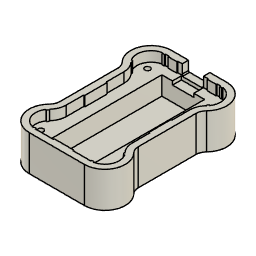
tiny-scarab-v0.2-enclosure (Autodesk Fusion 360 design; units mm, degrees)
Autodesk Fusion 360 part; units mm, degrees
sketch "board_cutout_1mm_offset" plane through (0, 0, 0) normal (0, 0, 1) x (1, 0, 0)
  line L0 (79.75, -21.495) -> (110.75, -21.495) construction
  arc A0 (79.75, -21.495) -> (74.3929, -34.2439) centre (79.75, -28.995) ccw construction
  arc A1 (77.25, -41.2424) -> (74.3929, -34.2439) centre (67.25, -41.2424) ccw construction
  line L1 (77.25, -41.2424) -> (77.25, -73.7476) construction
  arc A2 (74.3929, -80.7461) -> (77.25, -73.7476) centre (67.25, -73.7476) ccw construction
  arc A3 (74.3929, -80.7461) -> (79.75, -93.495) centre (79.75, -85.995) ccw construction
  line L2 (79.75, -93.495) -> (110.75, -93.495) construction
  arc A4 (110.75, -93.495) -> (116.1071, -80.7461) centre (110.75, -85.995) ccw construction
  arc A5 (113.25, -73.7476) -> (116.1071, -80.7461) centre (123.25, -73.7476) ccw construction
  line L3 (113.25, -41.2424) -> (113.25, -73.7476) construction
  arc A6 (116.1071, -34.2439) -> (113.25, -41.2424) centre (123.25, -41.2424) ccw construction
  arc A7 (116.1071, -34.2439) -> (110.75, -21.495) centre (110.75, -28.995) ccw construction
  arc A8 (76.75, -41.2424) -> (74.0357, -34.5938) centre (67.25, -41.2424) ccw
  arc A9 (78.3608, -21.1165) -> (73.1503, -33.5165) centre (79.75, -28.995) ccw
  arc A10 (117.3497, -33.5165) -> (112.1392, -21.1165) centre (110.75, -28.995) ccw
  arc A11 (116.4643, -34.5938) -> (113.75, -41.2424) centre (123.25, -41.2424) ccw
  arc A12 (113.75, -73.7476) -> (116.4643, -80.3962) centre (123.25, -73.7476) ccw
  arc A13 (112.1392, -93.8735) -> (117.3497, -81.4735) centre (110.75, -85.995) ccw
  arc A14 (73.1503, -81.4735) -> (78.3608, -93.8735) centre (79.75, -85.995) ccw
  arc A15 (74.0357, -80.3962) -> (76.75, -73.7476) centre (67.25, -73.7476) ccw
  line L4 (81.75, -20.995) -> (81.75, -21.495)
  line L5 (108.75, -21.495) -> (108.75, -20.995)
  line L6 (79.75, -20.995) -> (81.75, -20.995)
  line L7 (108.75, -20.995) -> (110.75, -20.995)
  line L8 (89.75, -93.995) -> (89.75, -93.495)
  line L9 (89.75, -93.495) -> (100.75, -93.495)
  line L10 (100.75, -93.495) -> (100.75, -93.995)
  line L11 (79.75, -93.995) -> (89.75, -93.995)
  line L12 (100.75, -93.995) -> (110.75, -93.995)
  line L13 (76.75, -51.2424) -> (77.25, -51.2424)
  line L14 (77.25, -51.2424) -> (77.25, -63.7476)
  line L15 (77.25, -63.7476) -> (76.75, -63.7476)
  line L16 (76.75, -41.2424) -> (76.75, -51.2424)
  line L17 (76.75, -63.7476) -> (76.75, -73.7476)
  line L18 (113.75, -51.2424) -> (113.25, -51.2424)
  line L19 (113.25, -51.2424) -> (113.25, -63.7476)
  line L20 (113.25, -63.7476) -> (113.75, -63.7476)
  line L21 (113.75, -41.2424) -> (113.75, -51.2424)
  line L22 (113.75, -63.7476) -> (113.75, -73.7476)
  line L23 (86.75, -21.495) -> (86.75, -20.995)
  line L24 (86.75, -20.995) -> (103.75, -20.995)
  line L25 (103.75, -20.995) -> (103.75, -21.495)
  line L26 (81.75, -21.495) -> (86.75, -21.495)
  line L27 (103.75, -21.495) -> (108.75, -21.495)
  arc A16 (116.1071, -34.2439) -> (116.9372, -33.2339) centre (110.75, -28.995) ccw
  line L28 (110.75, -28.995) -> (116.1071, -34.2439) construction
  line L29 (110.75, -28.995) -> (116.9372, -33.2339) construction
  line L30 (79.75, -28.995) -> (74.3929, -34.2439) construction
  arc A17 (73.5628, -33.2339) -> (74.3929, -34.2439) centre (79.75, -28.995) ccw
  line L31 (73.5628, -33.2339) -> (79.75, -28.995) construction
  line L32 (79.75, -85.995) -> (74.3929, -80.7461) construction
  arc A18 (74.3929, -80.7461) -> (73.5628, -81.7561) centre (79.75, -85.995) ccw
  line L33 (73.5628, -81.7561) -> (79.75, -85.995) construction
  line L34 (110.75, -85.995) -> (116.1071, -80.7461) construction
  arc A19 (116.9372, -81.7561) -> (116.1071, -80.7461) centre (110.75, -85.995) ccw
  line L35 (110.75, -85.995) -> (116.9372, -81.7561) construction
  line L36 (110.75, -85.995) -> (110.75, -93.495) construction
  arc A20 (110.75, -93.495) -> (112.0524, -93.3811) centre (110.75, -85.995) ccw
  line L37 (110.75, -85.995) -> (112.0524, -93.3811) construction
  line L38 (79.75, -85.995) -> (79.75, -93.495) construction
  arc A21 (78.4476, -93.3811) -> (79.75, -93.495) centre (79.75, -85.995) ccw
  line L39 (78.4476, -93.3811) -> (79.75, -85.995) construction
  line L40 (79.75, -28.995) -> (79.75, -21.495) construction
  arc A22 (79.75, -21.495) -> (78.4476, -21.6089) centre (79.75, -28.995) ccw
  line L41 (79.75, -28.995) -> (78.4476, -21.6089) construction
  line L42 (110.75, -28.995) -> (110.75, -21.495) construction
  arc A23 (112.0524, -21.6089) -> (110.75, -21.495) centre (110.75, -28.995) ccw
  line L43 (112.0524, -21.6089) -> (110.75, -28.995) construction
  line L44 (116.1071, -34.2439) -> (116.4643, -34.5938)
  line L45 (116.9372, -33.2339) -> (117.3497, -33.5165)
  line L46 (110.75, -21.495) -> (110.75, -20.995)
  line L47 (112.0524, -21.6089) -> (112.1392, -21.1165)
  line L48 (79.75, -21.495) -> (79.75, -20.995)
  line L49 (78.4476, -21.6089) -> (78.3608, -21.1165)
  line L50 (73.5628, -33.2339) -> (73.1503, -33.5165)
  line L51 (74.3929, -34.2439) -> (74.0357, -34.5938)
  line L52 (74.3929, -80.7461) -> (74.0357, -80.3962)
  line L53 (73.5628, -81.7561) -> (73.1503, -81.4735)
  line L54 (78.4476, -93.3811) -> (78.3608, -93.8735)
  line L55 (79.75, -93.495) -> (79.75, -93.995)
  line L56 (110.75, -93.495) -> (110.75, -93.995)
  line L57 (112.0524, -93.3811) -> (112.1392, -93.8735)
  line L58 (116.1071, -80.7461) -> (116.4643, -80.3962)
  line L59 (116.9372, -81.7561) -> (117.3497, -81.4735)
  dimension "d81" = 72
  dimension "d82" = 36
  dimension "d83" = 2
  dimension "d84" = 2
  dimension "d85" = 10
  dimension "d86" = 10
  dimension "d87" = 9.5
  dimension "d88" = 9.5
  dimension "d89" = 9.5
  dimension "d90" = 9.5
  dimension "d91" = 10
  dimension "d92" = 10
  dimension "d93" = 10
  dimension "d94" = 10
  dimension "d95" = 0.5
  dimension "d96" = 5
  dimension "d97" = 5
  dimension "d98" = 73
  dimension "d99" = 7.5
  dimension "d100" = 10
  dimension "d101" = 10
  dimension "d102" = 7.5
  dimension "d103" = 10
  dimension "d104" = 7.5
  dimension "d105" = 10
  dimension "d106" = 7.5
  dimension "d107" = 10
  dimension "d108" = 7.5
  dimension "d109" = 10
  dimension "d110" = 7.5
  dimension "d111" = 10
  dimension "d112" = 7.5
  dimension "d113" = 10
  dimension "d114" = 7.5
  constraint coincident L0 L4.end
  constraint perpendicular L0 L4
  constraint coincident L0 L5.start
  constraint coincident L5.end L6
  constraint perpendicular L5 L6
  constraint concentric A1 A8
  constraint concentric A0 A9
  constraint concentric A7 A10
  constraint concentric A6 A11
  constraint concentric A5 A12
  constraint concentric A4 A13
  constraint concentric A3 A14
  constraint concentric A2 A15
  constraint tangent A10 L6
  constraint tangent A9 L6
  constraint tangent A13 L11
  constraint tangent A14 L11
  constraint collinear L6 L7
  constraint coincident L2 L8.end
  constraint perpendicular L2 L8
  constraint coincident L2 L9.end
  constraint coincident L10.end L11
  constraint perpendicular L10 L11
  constraint collinear L11 L12
  constraint coincident L1 L13.end
  constraint perpendicular L1 L13
  constraint coincident L1 L14.end
  constraint perpendicular L13 L14
  constraint coincident L15.end L16
  constraint perpendicular L15 L16
  constraint collinear L16 L17
  constraint coincident L3 L18.end
  constraint perpendicular L3 L18
  constraint coincident L3 L19.end
  constraint perpendicular L18 L19
  constraint coincident L20.end L21
  constraint perpendicular L20 L21
  constraint collinear L21 L22
  constraint coincident L0 L23.start
  constraint perpendicular L23 L26
  constraint perpendicular L23 L24
  constraint coincident L0 L25.end
  constraint vertical L25
  constraint collinear L26 L27
  constraint coincident A7 A6.start
  constraint coincident A7 A16.end
  constraint coincident A6.start A7.start
  constraint coincident A7.centre A10.centre
  constraint coincident A0.centre A9.centre
  constraint coincident A0.end A1.end
  constraint coincident A0 A17.start
  constraint coincident A3.centre A14.centre
  constraint coincident A2.start A3.start
  constraint coincident A3 A18.end
  constraint coincident A4.centre A13.centre
  constraint coincident A4.end A5.end
  constraint coincident L2.end A4.start
  constraint coincident A4 A20.end
  constraint coincident A3.end L2.start
  constraint coincident L0.start A0.start
  constraint coincident L0.end A7.end
  constraint parallel L29 L45
  constraint parallel L28 L44
  constraint coincident A10 L7.end
  constraint parallel L43 L47
  constraint parallel L42 L46
  constraint coincident A9 L6.start
  constraint parallel L40 L48
  constraint parallel L41 L49
  constraint coincident A8 L51.end
  constraint parallel L30 L51
  constraint parallel L31 L50
  constraint coincident A15 L52.end
  constraint parallel L33 L53
  constraint parallel L32 L52
  constraint coincident A14 L11.start
  constraint parallel L38 L55
  constraint parallel L39 L54
  constraint coincident A13 L12.end
  constraint parallel L37 L57
  constraint parallel L36 L56
  constraint coincident A12 L58.end
  constraint parallel L34 L58
  constraint parallel L35 L59
  constraint coincident L7.end L46
  constraint coincident L6.start L48
  constraint coincident L11.start L55
  constraint coincident L12.end L56
  constraint coincident A12.end L58
  constraint coincident A15.start L52
  constraint coincident A8.end L51
  measures "d81" distance of L0 L2
  measures "d82" distance of L1 L3
  measures "d83" distance of L0.start L4
  measures "d84" horizontal distance of L0.end L5.end
  measures "d85" distance of A3.end L8
  measures "d86" distance of L2.end L10
  measures "d87" radius of A12
  measures "d88" radius of A15
  measures "d89" radius of A8
  measures "d90" radius of A11
  measures "d91" distance of L1.end L15
  measures "d92" distance of A1.start L13
  measures "d93" distance of L3.start L18
  measures "d94" distance of A5.start L20
  measures "d95" distance of L24 L27
  measures "d96" distance of L4.end L23
  measures "d97" distance of L5.start L25
  measures "d98" distance of L12 L24
  measures "d99" radius of A16
  measures "d100" angle of L28 L29
  measures "d101" angle of L30 L31
  measures "d102" radius of A17
  measures "d103" angle of L32 L33
  measures "d104" radius of A18
  measures "d105" angle of L34 L35
  measures "d106" radius of A19
  measures "d107" angle of L36 L37
  measures "d108" radius of A20
  measures "d109" angle of L38 L39
  measures "d110" radius of A21
  measures "d111" angle of L40 L41
  measures "d112" radius of A22
  measures "d113" angle of L42 L43
  measures "d114" radius of A23
sketch "block_2mm_offset" plane through (0, 0, 0) normal (0, 0, 1) x (1, 0, 0)
  line L0 (85.25, -28.495) -> (105.25, -28.495) construction
  line L1 (85.25, -86.495) -> (85.25, -28.495) construction
  line L2 (105.25, -86.495) -> (85.25, -86.495) construction
  line L3 (105.25, -28.495) -> (105.25, -86.495) construction
  line L4 (107.25, -88.495) -> (83.25, -88.495)
  line L5 (83.25, -88.495) -> (83.25, -26.495)
  line L6 (83.25, -26.495) -> (107.25, -26.495)
  line L7 (107.25, -26.495) -> (107.25, -88.495)
  dimension "d2" = -2
sketch "sketch 7142" plane through (0, 0, 0) normal (0, 0, 1) x (1, 0, 0)
  line L0 (79.75, -21.495) -> (110.75, -21.495) construction
  arc A0 (79.75, -21.495) -> (74.3929, -34.2439) centre (79.75, -28.995) ccw construction
  arc A1 (77.25, -41.2424) -> (74.3929, -34.2439) centre (67.25, -41.2424) ccw construction
  line L1 (77.25, -41.2424) -> (77.25, -73.7476) construction
  arc A2 (74.3929, -80.7461) -> (77.25, -73.7476) centre (67.25, -73.7476) ccw construction
  arc A3 (74.3929, -80.7461) -> (79.75, -93.495) centre (79.75, -85.995) ccw construction
  line L2 (79.75, -93.495) -> (110.75, -93.495) construction
  arc A4 (110.75, -93.495) -> (116.1071, -80.7461) centre (110.75, -85.995) ccw construction
  arc A5 (113.25, -73.7476) -> (116.1071, -80.7461) centre (123.25, -73.7476) ccw construction
  line L3 (113.25, -41.2424) -> (113.25, -73.7476) construction
  arc A6 (116.1071, -34.2439) -> (113.25, -41.2424) centre (123.25, -41.2424) ccw construction
  arc A7 (116.1071, -34.2439) -> (110.75, -21.495) centre (110.75, -28.995) ccw construction
  arc A8 (117.25, -73.7476) -> (118.9643, -77.9467) centre (123.25, -73.7476) ccw
  arc A9 (110.75, -97.495) -> (118.9643, -77.9467) centre (110.75, -85.995) ccw
  line L4 (79.75, -97.495) -> (110.75, -97.495)
  arc A10 (71.5357, -77.9467) -> (79.75, -97.495) centre (79.75, -85.995) ccw
  arc A11 (71.5357, -77.9467) -> (73.25, -73.7476) centre (67.25, -73.7476) ccw
  line L5 (73.25, -41.2424) -> (73.25, -73.7476)
  arc A12 (73.25, -41.2424) -> (71.5357, -37.0433) centre (67.25, -41.2424) ccw
  arc A13 (79.75, -17.495) -> (71.5357, -37.0433) centre (79.75, -28.995) ccw
  line L6 (79.75, -17.495) -> (110.75, -17.495)
  arc A14 (118.9643, -37.0433) -> (110.75, -17.495) centre (110.75, -28.995) ccw
  arc A15 (118.9643, -37.0433) -> (117.25, -41.2424) centre (123.25, -41.2424) ccw
  line L7 (117.25, -41.2424) -> (117.25, -73.7476)
extrude "Extrude1" add sketch "sketch 7142" along normal blind 20
extrude "Extrude2" cut sketch "board_cutout_1mm_offset" against normal blind 5.6 from surface at 20
extrude "Extrude3" cut sketch "block_2mm_offset" against normal blind 10.4 from surface at 14.4
sketch "sketch 7468" plane through (0, 0, 0) normal (0, 0, 1) x (1, 0, 0)
  circle A0 centre (76.25, -27.495) radius 1.5 construction
  circle A1 centre (114.25, -27.495) radius 1.5 construction
  circle A2 centre (76.25, -87.495) radius 1.5 construction
  circle A3 centre (114.25, -87.495) radius 1.5 construction
  circle A4 centre (76.25, -27.495) radius 3
  circle A5 centre (114.25, -27.495) radius 3
  circle A6 centre (76.25, -87.495) radius 3
  circle A7 centre (114.25, -87.495) radius 3
extrude "Extrude5" cut sketch "sketch 7468" along normal blind 8.2
sketch "usb_top" plane through (0, 0, 0) normal (0, 0, 1) x (1, 0, 0)
  line L0 (90.75, -28.995) -> (90.75, -21.495) construction
  line L1 (90.75, -21.495) -> (99.75, -21.495)
  line L2 (99.75, -21.495) -> (99.75, -28.995) construction
  line L3 (99.75, -28.995) -> (90.75, -28.995) construction
  line L4 (89.25, -21.495) -> (101.25, -21.495)
  line L5 (101.25, -21.495) -> (101.25, -29.995)
  line L6 (101.25, -29.995) -> (89.25, -29.995)
  line L7 (89.25, -29.995) -> (89.25, -21.495)
  dimension "d14" = 12
  dimension "d15" = 1
  dimension "d16" = 1.5
  dimension "d17" = 1.5
  constraint horizontal L4
  constraint vertical L5
  constraint horizontal L6
  constraint vertical L7
  constraint midpoint L1 L4
  measures "d14" distance of L5 L7
  measures "d15" distance of L3 L6
  measures "d16" distance of L2 L5
  measures "d17" distance of L0 L7
extrude "Extrude6" cut sketch "usb_top" against normal blind 2 from surface at 14.4
sketch "usb_front_drawing" plane through (0, -17.495, 0) normal (0, 1, 0) x (-1, 0, 0)
  line L0 (-101.25, 20.58) -> (-89.25, 20.58)
  line L1 (-89.25, 20.58) -> (-89.25, 14.4)
  line L2 (-89.25, 14.4) -> (-101.25, 14.4)
  line L3 (-101.25, 14.4) -> (-101.25, 20.58)
  line L4 (-101.25, 14.4) -> (-101.25, 12.4)
  line L5 (-83.25, 14.4) -> (-83.25, 4) construction
  line L6 (-107.25, 14.4) -> (-107.25, 4) construction
  line L7 (-95.25, 20) -> (-95.25, 0) construction
  line L8 (-79.75, 16) -> (-110.75, 16) construction
  line L9 (-98.92, 19.16) -> (-91.58, 19.16)
  line L10 (-90.78, 18.36) -> (-90.78, 16.8)
  line L11 (-91.58, 16) -> (-98.92, 16)
  line L12 (-99.72, 16.8) -> (-99.72, 18.36)
  line L13 (-98.595, 18.18) -> (-91.905, 18.18)
  line L14 (-91.905, 18.18) -> (-91.905, 16.98)
  line L15 (-91.905, 16.98) -> (-98.595, 16.98)
  line L16 (-98.595, 16.98) -> (-98.595, 18.18)
  arc A0 (-98.92, 19.16) -> (-99.72, 18.36) centre (-98.92, 18.36) ccw
  arc A1 (-90.78, 18.36) -> (-91.58, 19.16) centre (-91.58, 18.36) ccw
  arc A2 (-91.08, 18.36) -> (-91.58, 18.86) centre (-91.58, 18.36) ccw
  line L17 (-98.92, 18.86) -> (-91.58, 18.86)
  arc A3 (-98.92, 18.86) -> (-99.42, 18.36) centre (-98.92, 18.36) ccw
  line L18 (-99.42, 16.8) -> (-99.42, 18.36)
  arc A4 (-99.42, 16.8) -> (-98.92, 16.3) centre (-98.92, 16.8) ccw
  line L19 (-91.58, 16.3) -> (-98.92, 16.3)
  arc A5 (-91.58, 16.3) -> (-91.08, 16.8) centre (-91.58, 16.8) ccw
  line L20 (-91.08, 18.36) -> (-91.08, 16.8)
  line L21 (-99.72, 16.8) -> (-99.72, 14.1)
  line L22 (-99.42, 14.1) -> (-99.42, 16)
  line L23 (-99.72, 14.1) -> (-99.42, 14.1)
  line L24 (-90.78, 16.8) -> (-90.78, 14.1)
  line L25 (-91.08, 14.1) -> (-91.08, 16)
  line L26 (-91.08, 14.1) -> (-90.78, 14.1)
  line L27 (-99.42, 16) -> (-98.92, 16)
  line L28 (-91.08, 16) -> (-91.58, 16)
  line L29 (-98.595, 17.58) -> (-91.905, 17.58) construction
  line L30 (-110.75, 14.4) -> (-79.75, 14.4)
  line L31 (-110.75, 0) -> (-79.75, 0)
  line L32 (-79.75, 0) -> (-79.75, 20)
  line L33 (-79.75, 20) -> (-110.75, 20)
  line L34 (-110.75, 20) -> (-110.75, 0)
  dimension "d21" = 12
  dimension "d25" = 24
  dimension "d26" = 12
  dimension "d29" = 4.47
  dimension "d30" = 8.94
  dimension "d31" = 3.16
  dimension "d32" = 6.69
  dimension "d33" = 3.345
  dimension "d34" = 1.2
  dimension "d35" = 0.98
  dimension "d36" = 0.98
  dimension "d37" = 0.8
  dimension "d39" = 0.8
  dimension "d42" = 8.34
  dimension "d43" = 0.3
  dimension "d45" = 0.3
  dimension "d47" = 0.5
  dimension "d48" = 0.5
  dimension "d49" = 0.6
  dimension "d50" = 3
  dimension "d51" = 3.18
  dimension "d63" = 1.6
  constraint horizontal L0
  constraint vertical L1
  constraint horizontal L2
  constraint vertical L3
  constraint collinear L3 L4
  constraint vertical L7
  constraint horizontal L9
  constraint vertical L10
  constraint horizontal L11
  constraint vertical L12
  constraint collinear L8 L11
  constraint horizontal L13
  constraint vertical L14
  constraint horizontal L15
  constraint vertical L16
  constraint tangent L9 A0
  constraint tangent L12 A0
  constraint tangent L9 A1
  constraint tangent L10 A1
  constraint coincident L8 L22.end
  constraint perpendicular L8 L22
  constraint perpendicular L22 L23
  constraint coincident L8 L25.end
  constraint perpendicular L8 L25
  constraint perpendicular L24 L26
  constraint concentric A1 A2
  constraint concentric A0 A3
  constraint tangent L18 A4
  constraint tangent A2 L20
  constraint tangent A2 L17
  constraint tangent L17 A3
  constraint tangent A5 L20
  constraint tangent A3 L18
  constraint tangent A4 L19
  constraint tangent L19 A5
  constraint coincident L16 L29.start
  constraint coincident L14 L29.end
  constraint perpendicular L14 L29
  measures "d21" distance of L1 L3
  measures "d25" distance of L5 L6
  measures "d26" distance of L5 L7
  measures "d29" distance of L7 L10
  measures "d30" distance of L10 L12
  measures "d31" distance of L9 L11
  measures "d32" distance of L14 L16
  measures "d33" distance of L7 L14
  measures "d34" distance of L13 L15
  measures "d35" distance of L8 L15
  measures "d36" distance of L9 L13
  measures "d37" radius of A0
  measures "d39" radius of A1
  measures "d42" distance of L18 L20
  measures "d43" distance of L21 L22
  measures "d45" distance of L24 L25
  measures "d47" radius of A5
  measures "d48" radius of A4
  measures "d49" distance of L15 L29
  measures "d50" distance of L0 L29
  measures "d51" distance of L2 L29
  measures "d63" distance of L8 L30
sketch "usb_front_cutout" plane through (0, -17.495, 0) normal (0, 1, 0) x (-1, 0, 0)
  line L0 (-101.25, 20.58) -> (-89.25, 20.58) construction
  line L1 (-101.25, 14.4) -> (-101.25, 20.58) construction
  line L2 (-89.25, 14.4) -> (-101.25, 14.4) construction
  line L3 (-89.25, 20.58) -> (-89.25, 14.4) construction
  line L4 (-100.67, 20.58) -> (-89.83, 20.58)
  line L5 (-89.25, 20) -> (-89.25, 14.98)
  line L6 (-89.83, 14.4) -> (-100.67, 14.4)
  line L7 (-101.25, 14.98) -> (-101.25, 20)
  arc A0 (-100.67, 20.58) -> (-101.25, 20) centre (-100.67, 20) ccw
  arc A1 (-101.25, 14.98) -> (-100.67, 14.4) centre (-100.67, 14.98) ccw
  arc A2 (-89.25, 20) -> (-89.83, 20.58) centre (-89.83, 20) ccw
  arc A3 (-89.83, 14.4) -> (-89.25, 14.98) centre (-89.83, 14.98) ccw
  line L8 (-110.75, 0) -> (-79.75, 0)
  line L9 (-79.75, 0) -> (-79.75, 20)
  line L10 (-79.75, 20) -> (-110.75, 20)
  line L11 (-110.75, 20) -> (-110.75, 0)
  dimension "d52" = 0.58
  dimension "d53" = 0.58
  dimension "d54" = 0.58
  dimension "d55" = 0.58
  dimension "d58" = 6.18
  dimension "d59" = 12
  dimension "d60" = 0.58
  constraint horizontal L4
  constraint vertical L5
  constraint horizontal L6
  constraint vertical L7
  constraint tangent L4 A0
  constraint tangent L7 A0
  constraint tangent L6 A1
  constraint tangent L7 A1
  constraint tangent L4 A2
  constraint tangent L5 A2
  constraint tangent L5 A3
  constraint tangent L6 A3
  constraint collinear L2 L6
  constraint collinear L1 L7
  constraint collinear L3 L5
  constraint collinear L0 L4
  measures "d52" radius of A0
  measures "d53" radius of A1
  measures "d54" radius of A2
  measures "d55" radius of A3
  measures "d58" distance of L4 L6
  measures "d59" distance of L5 L7
  measures "d60" radius of A0
extrude "Extrude7" cut sketch "usb_front_cutout" against normal up to surface (3.5 mm away) contours L4 A0 A2 L10 | L5 L6 L7 A1 A3 L10
sketch "screw_holes_3mm" plane through (0, 0, 0) normal (0, 0, 1) x (1, 0, 0)
  circle A0 centre (76.25, -27.495) radius 1.5 construction
  circle A1 centre (114.25, -27.495) radius 1.5 construction
  circle A2 centre (76.25, -87.495) radius 1.5 construction
  circle A3 centre (114.25, -87.495) radius 1.5 construction
  circle A4 centre (76.25, -27.495) radius 1.5
  circle A5 centre (114.25, -27.495) radius 1.5
  circle A6 centre (76.25, -87.495) radius 1.5
  circle A7 centre (114.25, -87.495) radius 1.5
  dimension "d64" = 3
  dimension "d65" = 3
  dimension "d66" = 3
  dimension "d67" = 3
  constraint concentric A0 A4
  constraint concentric A1 A5
  constraint concentric A2 A6
  constraint concentric A3 A7
  measures "d64" diameter of A4
  measures "d65" diameter of A5
  measures "d66" diameter of A6
  measures "d67" diameter of A7
extrude "Extrude8" cut sketch "screw_holes_3mm" along normal through all
chamfer "Chamfer1" distance 1.5 angle 45 1 edges at (112.8515, -88.0374, 8.2)
chamfer "Chamfer2" distance 1.5 angle 45 1 edges at (112.8515, -28.0374, 8.2)
chamfer "Chamfer3" distance 1.5 angle 45 1 edges at (74.8515, -28.0374, 8.2)
chamfer "Chamfer4" distance 1.5 angle 45 1 edges at (74.8515, -88.0374, 8.2)
